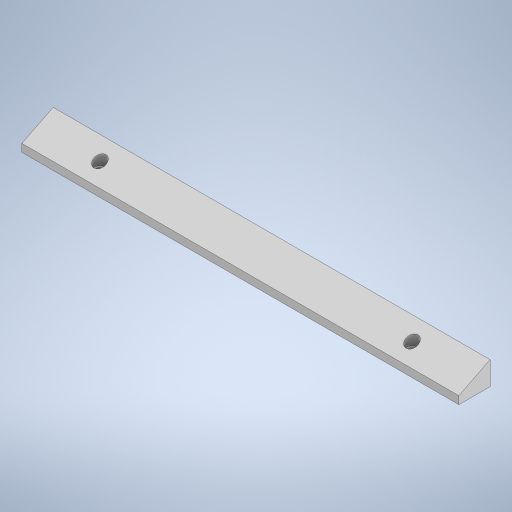
# Autodesk Inventor part: paw shelf_v03
Saved by Autodesk Inventor 2023 (Build 270158000, 158)
## iProperties
Created: 2023-02-22
Part Number: paw shelf_v03
Material: Generic
Document SubType Name: Modeling
Designer: Akramilab
Density: 1 g/cm^3
Appearance: Default
Author: Akramilab
Autodesk Inventor part; units mm, degrees
ref_plane "YZ Plane" through (0, 0, 0) normal (1, 0, 0) x (0, 1, 0)
ref_plane "XZ Plane" through (0, 0, 0) normal (0, 1, 0) x (-1, 0, 0)
ref_plane "XY Plane" through (0, 0, 0) normal (0, 0, 1) x (1, 0, 0)
sketch "Sketch1" plane through (0, 0, 0) normal (0, 0, 1) x (1, 0, 0)
  line L0 (140, 5) -> (-140, 5)
  line L1 (-140, 5) -> (-140, -5)
  line L2 (-140, -5) -> (140, -5)
  line L3 (140, -5) -> (140, 5)
  line L4 (140, 5) -> (-140, -5) construction
  line L5 (-140, 5) -> (140, -5) construction
  point P0 (0, 0)
  dimension "d0" = 280
  dimension "d1" = 10
  constraints: 12 end point, 2 midpoint, 2 parallel, 1 horizontal, 1 perpendicular
  measures "d0" distance of L2.end L1.end
  measures "d1" distance of L1.end L0.end
extrude "Extrusion1" add sketch "Sketch1" along normal blind 20
sketch "Sketch6" plane through (-140, -5, 0) normal (0, -1, 0) x (1, 0, 0)
  line L0 (0, 0) -> (0, 20) projected
  line L1 (0, 0) -> (280, 0) projected
  line L2 (0, 20) -> (280, 20)
  line L3 (280, 20) -> (280, 0)
  line L4 (280, 0) -> (0, 0)
  line L5 (0, 0) -> (0, 20)
  point P0 (140, 0)
  constraints: 8 end point, 2 parallel, 1 horizontal, 1 perpendicular
extrude "Extrusion4" add sketch "Sketch6" along normal blind 5
sketch "Sketch7" plane through (-140, -10, 0) normal (0, -1, 0) x (1, 0, 0)
  point P0 (140, 0)
sketch "Sketch8" plane through (-140, -10, 0) normal (0, -1, 0) x (1, 0, 0)
  circle A0 centre (40, 10) radius 2.1 projected
  circle A1 centre (40, 10) radius 2.25
  circle A2 centre (240, 10) radius 2.25
  line L0 (280, 20) -> (0, 20) projected
  line L1 (0, 20) -> (0, 0) projected
  point P0 (140, 0)
  dimension "d23" = 4.5
  dimension "d24" = 4.5
  dimension "d35" = 200
  dimension "d36" = 10
  dimension "d37" = 10
  dimension "d38" = 40
  constraints: 2 centre point, 1 coincident
  measures "d23" diameter of A1
  measures "d24" diameter of A2
  measures "d35" distance of A2.centre A1.centre
  measures "d36" distance from line of A1.centre L0
  measures "d37" distance from line of L0 A2.centre
  measures "d38" distance from line of A1.centre L1
extrude "Extrusion5" cut sketch "Sketch8" against normal through all contours A0 | A1 | A2
sketch "Sketch9" plane through (-140, 5, 0) normal (0, 1, 0) x (1, 0, 0)
  circle A0 centre (40, -10) radius 2.25 projected
  circle A1 centre (40, -10) radius 3.75
  circle A2 centre (240, -10) radius 2.25 projected
  circle A3 centre (240, -10) radius 3.75
  point P0 (140, 0)
  dimension "d27" = 7.5
  dimension "d28" = 7.5
  constraints: 2 centre point, 2 coincident
  measures "d27" diameter of A1
  measures "d28" diameter of A3
extrude "Extrusion6" cut sketch "Sketch9" against normal blind 10 contours A0 | A1 | A2 | A3
sketch "Sketch10" plane through (-140, 5, 0) normal (-1, 0, 0) x (0, 0, 1)
  line L0 (0, 0) -> (20, 0) projected
  line L1 (20, 0) -> (20, -10)
  line L2 (20, 0) -> (20, -15) projected
  line L3 (20, 0) -> (30, 0) construction
  line L4 (0, 0) -> (0, -15) projected
  line L5 (20, -10) -> (0, 0)
  line L6 (0, 0) -> (20, 0)
  point P0 (0, -5)
  dimension "d31" = 10
  dimension "d32" = 90
  constraints: 8 end point, 2 perpendicular, 1 collinear, 1 horizontal
  measures "d31" distance of L0.end L1.end
  measures "d32" angle of L1 L3
extrude "Extrusion7" cut sketch "Sketch10" against normal through all
equation "\"d24\" = d23"
equation "\"d28\" = d27"
body "Solid1"
